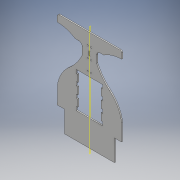
# Autodesk Inventor part: 底盤新
Saved by Autodesk Inventor 2019 (Build 230136000, 136)
## iProperties
Created: 2020-03-19
Part Number: 底盤新
Material: 一般
Document SubType Name: Modeling
Designer: 吳昇峻
Density: 1 g/cm^3
Appearance: 預設
Author: 吳昇峻
Autodesk Inventor part; units mm, degrees
ref_plane "YZ Plane" through (0, 0, 0) normal (1, 0, 0) x (0, 1, 0)
ref_plane "XZ Plane" through (0, 0, 0) normal (0, 1, 0) x (-1, 0, 0)
ref_plane "XY Plane" through (0, 0, 0) normal (0, 0, 1) x (1, 0, 0)
sketch "草圖1" plane through (0, 0, 0) normal (0, 1, 0) x (-1, 0, 0)
  line L0 (413.5961, 122.1998) -> (413.5961, 137.1998)
  arc A0 (413.5961, 137.1998) -> (408.5961, 142.1998) centre (408.5961, 137.1998) ccw
  line L1 (233.5961, 122.1998) -> (233.5961, 137.1998)
  line L2 (238.5961, 142.1998) -> (408.5961, 142.1998)
  line L3 (303.5961, 77.1998) -> (303.5961, 97.1998)
  arc A1 (303.5961, 97.1998) -> (293.5961, 107.1998) centre (293.5961, 97.1998) ccw
  line L4 (293.5961, 107.1998) -> (283.5961, 107.1998)
  line L5 (343.5961, 77.1998) -> (343.5961, 97.1998)
  arc A2 (353.5961, 107.1998) -> (343.5961, 97.1998) centre (353.5961, 97.1998) ccw
  line L6 (353.5961, 107.1998) -> (363.5961, 107.1998)
  line L7 (233.5961, 137.1998) -> (233.5961, 122.1998)
  arc A3 (238.5961, 142.1998) -> (233.5961, 137.1998) centre (238.5961, 137.1998) ccw
  arc A4 (283.5961, 107.1998) -> (233.5961, 122.1998) centre (233.5961, 31.3665) ccw
  arc A5 (413.5961, 122.1998) -> (363.5961, 107.1998) centre (413.5961, 31.3665) ccw
  line L8 (356.5961, 34.1998) -> (290.5961, 34.1998)
  line L9 (290.5961, 24.1998) -> (290.5961, 4.1998)
  line L10 (290.5961, -5.8002) -> (290.5961, -25.8002)
  line L11 (290.5961, -35.8002) -> (290.5961, -55.8002)
  line L12 (290.5961, -65.8002) -> (356.5961, -65.8002)
  line L13 (263.5961, -138.8002) -> (383.5961, -138.8002)
  line L14 (233.6991, -53.0551) -> (233.6991, -78.8002)
  line L15 (413.5961, -78.8002) -> (413.4932, -53.0551)
  arc A6 (267.2809, 29.4379) -> (303.5961, 77.1998) centre (176.7496, 135.9594) ccw
  arc A7 (267.2809, 29.4379) -> (233.6991, -32.0184) centre (330.5999, -45.0649) ccw
  arc A8 (343.5961, 77.1998) -> (379.9114, 29.4379) centre (470.4427, 135.9594) ccw
  arc A9 (413.4932, -32.0184) -> (379.9114, 29.4379) centre (316.5923, -45.0649) ccw
  line L16 (413.4932, -32.0184) -> (413.4932, -53.0551)
  line L17 (233.6991, -32.0184) -> (233.6991, -53.0551)
  line L18 (290.5961, -55.8002) -> (290.5961, -35.8002)
  line L19 (290.5961, -25.8002) -> (290.5961, -5.8002)
  line L20 (290.5961, 4.1998) -> (290.5961, 24.1998)
  line L21 (290.5961, 34.1998) -> (287.5961, 34.1998)
  line L22 (287.5961, -65.8002) -> (290.5961, -65.8002)
  line L23 (287.5961, 4.1998) -> (290.5961, 4.1998)
  line L24 (290.5961, 4.1998) -> (290.5961, 24.1998)
  line L25 (290.5961, 24.1998) -> (287.5961, 24.1998)
  line L26 (290.5961, -5.8002) -> (287.5961, -5.8002)
  line L27 (287.5961, -25.8002) -> (290.5961, -25.8002)
  line L28 (290.5961, -25.8002) -> (290.5961, -5.8002)
  line L29 (290.5961, -35.8002) -> (287.5961, -35.8002)
  line L30 (287.5961, -55.8002) -> (290.5961, -55.8002)
  line L31 (290.5961, -55.8002) -> (290.5961, -35.8002)
  line L32 (287.5961, 34.1998) -> (286.5961, 34.1998)
  line L33 (286.5961, 34.1998) -> (286.5961, 24.1998)
  line L34 (286.5961, 4.1998) -> (286.5961, -5.8002)
  line L35 (286.5961, -25.8002) -> (286.5961, -35.8002)
  line L36 (286.5961, -55.8002) -> (286.5961, -65.8002)
  line L37 (286.5961, -65.8002) -> (287.5961, -65.8002)
  line L38 (287.5961, 24.1998) -> (286.5961, 24.1998)
  line L39 (287.5961, 4.1998) -> (286.5961, 4.1998)
  line L40 (287.5961, -5.8002) -> (286.5961, -5.8002)
  line L41 (287.5961, -25.8002) -> (286.5961, -25.8002)
  line L42 (287.5961, -35.8002) -> (286.5961, -35.8002)
  line L43 (287.5961, -55.8002) -> (286.5961, -55.8002)
  line L44 (356.5961, 24.1998) -> (356.5961, 4.1998)
  line L45 (356.5961, -5.8002) -> (356.5961, -25.8002)
  line L46 (356.5961, -35.8002) -> (356.5961, -55.8002)
  line L47 (356.5961, -55.8002) -> (356.5961, -35.8002)
  line L48 (356.5961, -25.8002) -> (356.5961, -5.8002)
  line L49 (356.5961, 4.1998) -> (356.5961, 24.1998)
  line L50 (356.5961, 34.1998) -> (359.5961, 34.1998)
  line L51 (359.5961, -65.8002) -> (356.5961, -65.8002)
  line L52 (359.5961, 4.1998) -> (356.5961, 4.1998)
  line L53 (356.5961, 4.1998) -> (356.5961, 24.1998)
  line L54 (356.5961, 24.1998) -> (359.5961, 24.1998)
  line L55 (356.5961, -5.8002) -> (359.5961, -5.8002)
  line L56 (359.5961, -25.8002) -> (356.5961, -25.8002)
  line L57 (356.5961, -25.8002) -> (356.5961, -5.8002)
  line L58 (356.5961, -35.8002) -> (359.5961, -35.8002)
  line L59 (359.5961, -55.8002) -> (356.5961, -55.8002)
  line L60 (356.5961, -55.8002) -> (356.5961, -35.8002)
  line L61 (359.5961, 34.1998) -> (360.5961, 34.1998)
  line L62 (360.5961, 34.1998) -> (360.5961, 24.1998)
  line L63 (360.5961, 4.1998) -> (360.5961, -5.8002)
  line L64 (360.5961, -25.8002) -> (360.5961, -35.8002)
  line L65 (360.5961, -55.8002) -> (360.5961, -65.8002)
  line L66 (360.5961, -65.8002) -> (359.5961, -65.8002)
  line L67 (359.5961, 24.1998) -> (360.5961, 24.1998)
  line L68 (359.5961, 4.1998) -> (360.5961, 4.1998)
  line L69 (359.5961, -5.8002) -> (360.5961, -5.8002)
  line L70 (359.5961, -25.8002) -> (360.5961, -25.8002)
  line L71 (359.5961, -35.8002) -> (360.5961, -35.8002)
  line L72 (359.5961, -55.8002) -> (360.5961, -55.8002)
  line L73 (323.5961, 97.1998) -> (325.0961, 97.1998)
  line L74 (325.0961, 97.1998) -> (325.0961, 89.1998)
  line L75 (325.0961, 85.1998) -> (322.0961, 85.1998)
  line L76 (322.0961, 89.1998) -> (322.0961, 97.1998)
  line L77 (322.0961, 97.1998) -> (323.5961, 97.1998)
  line L78 (322.0961, 85.1998) -> (322.0961, 89.1998)
  line L79 (325.0961, 85.1998) -> (325.0961, 89.1998)
  line L80 (323.5961, 77.1998) -> (408.5961, 77.1998) construction
  line L81 (323.5961, 77.1998) -> (238.5961, 77.1998) construction
  line L82 (408.5961, 107.1998) -> (393.5961, 107.1998) construction
  line L83 (393.5961, 107.1998) -> (393.5961, 47.1998) construction
  line L84 (393.5961, 47.1998) -> (423.5961, 47.1998) construction
  line L85 (423.5961, 47.1998) -> (423.5961, 107.1998) construction
  line L86 (423.5961, 107.1998) -> (408.5961, 107.1998) construction
  line L87 (238.5961, 107.1998) -> (253.5961, 107.1998) construction
  line L88 (253.5961, 107.1998) -> (253.5961, 47.1998) construction
  line L89 (253.5961, 47.1998) -> (223.5961, 47.1998) construction
  line L90 (223.5961, 47.1998) -> (223.5961, 107.1998) construction
  line L91 (223.5961, 107.1998) -> (238.5961, 107.1998) construction
  line L92 (253.5961, 77.1998) -> (257.5961, 77.1998) construction
  line L93 (257.5961, 77.1998) -> (257.5961, 82.1998) construction
  line L94 (393.5961, 77.1998) -> (389.5961, 77.1998) construction
  line L95 (389.5961, 77.1998) -> (389.5961, 82.1998) construction
  line L96 (257.5961, 77.1998) -> (261.5961, 77.1998) construction
  line L97 (389.5961, 77.1998) -> (385.5961, 77.1998)
  line L98 (261.5961, 77.1998) -> (271.5961, 77.1998)
  line L99 (271.5961, 77.1998) -> (318.5808, 60.0988) construction
  line L100 (271.5961, 77.1998) -> (318.5808, 94.3008) construction
  line L101 (385.5961, 77.1998) -> (375.5961, 77.1998)
  line L102 (375.5961, 77.1998) -> (328.6115, 94.3008) construction
  line L103 (375.5961, 77.1998) -> (328.6115, 60.0988) construction
  line L104 (261.5961, 77.1998) -> (274.2452, 39.2525) construction
  line L105 (274.2452, 39.2525) -> (372.947, 39.2525) construction
  line L106 (372.947, 39.2525) -> (385.5961, 77.1998) construction
  line L107 (323.5961, -108.8002) -> (408.5961, -108.8002) construction
  line L108 (323.5961, -108.8002) -> (238.5961, -108.8002) construction
  line L109 (423.5961, -108.8002) -> (423.5961, -78.8002) construction
  line L110 (423.5961, -78.8002) -> (393.5961, -78.8002)
  line L111 (393.5961, -78.8002) -> (393.5961, -138.8002)
  line L112 (393.5961, -138.8002) -> (423.5961, -138.8002) construction
  line L113 (423.5961, -138.8002) -> (423.5961, -108.8002) construction
  line L114 (223.5961, -108.8002) -> (223.5961, -78.8002) construction
  line L115 (223.5961, -78.8002) -> (253.5961, -78.8002)
  line L116 (253.5961, -78.8002) -> (253.5961, -138.8002)
  line L117 (253.5961, -138.8002) -> (223.5961, -138.8002) construction
  line L118 (223.5961, -138.8002) -> (223.5961, -108.8002) construction
  line L119 (393.5961, -138.8002) -> (383.5961, -138.8002)
  line L120 (263.5961, -138.8002) -> (253.5961, -138.8002)
  line L121 (318.5808, 94.3008) -> (318.5808, 108.3008) construction
  line L122 (328.6115, 94.3008) -> (328.6115, 108.3008) construction
  line L123 (328.6115, 60.0988) -> (328.6115, 46.0988) construction
  line L124 (318.5808, 60.0988) -> (318.5808, 46.0988) construction
  circle A10 centre (328.6115, 108.3008) radius 1.8
  circle A11 centre (318.5808, 108.3008) radius 1.8
  circle A12 centre (328.6115, 46.0988) radius 1.8
  circle A13 centre (318.5808, 46.0988) radius 1.8
  circle A14 centre (318.5808, 77.1998) radius 1.8
  circle A15 centre (328.6115, 77.1998) radius 1.8
  point P0 (0, 0)
  dimension "d0" = 14
  dimension "d1" = 14
  dimension "d2" = 14
  dimension "d3" = 3.6
  dimension "d4" = 3.6
  dimension "d5" = 3.6
  dimension "d6" = 3.6
  dimension "d7" = 3.6
  dimension "d8" = 3.6
  constraints: 250 end point, 20 point on circle, 16 centre point, 14 point on line, 4 coincident, 4 vertical, 2 midpoint, 1 collinear, 1 horizontal
  measures "d0" distance of L100.end L121.end
  measures "d1" distance of L102.end L122.end
  measures "d2" distance of L103.end L123.end
  measures "d3" diameter of A10
  measures "d4" diameter of A11
  measures "d5" diameter of A12
  measures "d6" diameter of A13
  measures "d7" diameter of A14
  measures "d8" diameter of A15
extrude "擠出1" add sketch "草圖1" along normal blind 3
ref_plane "Work Plane1" through (-323.5961, 0, 97.1998) normal (1, 0, 0) x (0, 0, -1)
